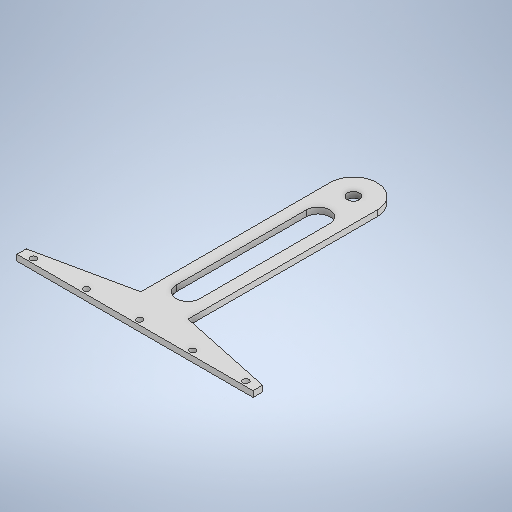
# Autodesk Inventor part: 03A
Saved by Autodesk Inventor 2025.1 (Build 291241000, 241)
## iProperties
Created: 2024-09-17
Part Number: 03A
Material: Generisch
Document SubType Name: Modeling
Designer: ffogue
Density: 1 g/cm^3
Appearance: Vorgabe
Author: ffogue
Autodesk Inventor part; units mm, degrees
ref_plane "YZ Plane" through (0, 0, 0) normal (1, 0, 0) x (0, 1, 0)
ref_plane "XZ Plane" through (0, 0, 0) normal (0, 1, 0) x (-1, 0, 0)
ref_plane "XY Plane" through (0, 0, 0) normal (0, 0, 1) x (1, 0, 0)
sketch "Sketch1" plane through (0, 0, 0) normal (0, 0, 1) x (1, 0, 0)
  line L0 (0, 0) -> (0, 91.5348) construction
  line L1 (-93.5855, 0) -> (93.5855, 0) construction
  arc A0 (20, 160) -> (-20, 160) centre (0, 160) ccw
  line L2 (-20, 160) -> (-20, 0)
  line L3 (-20, 0) -> (-100, -17)
  line L4 (-100, -17) -> (-100, -25)
  line L5 (-100, -25) -> (100, -25)
  line L6 (100, -25) -> (100, -17)
  line L7 (20, 160) -> (20, 0)
  line L8 (20, 0) -> (100, -17)
  dimension "d0" = 20
  dimension "d1" = 185
  dimension "d2" = 8
  dimension "d3" = 25
  dimension "d4" = 200
  constraints: 18 end point, 3 parallel, 3 perpendicular, 2 point on circle, 2 point on line, 2 tangent, 1 centre point, 1 horizontal, 1 midpoint, 1 vertical, 1 vertical alignment, 1 other
  measures "d0" radius of A0
  measures "d1" distance from line of L5 A0.centre
  measures "d2" distance of L3.end L4.end
  measures "d3" distance from line of L5 L2.end
  measures "d4" distance of L4.end L5.end
extrude "Extrusion1" add sketch "Sketch1" against normal blind 5
sketch "Sketch2" plane through (0, 0, 0) normal (0, 0, 1) x (1, 0, 0)
  line L0 (0, 20) -> (0, 130) construction
  line L1 (10, 20) -> (10, 130)
  line L2 (-10, 130) -> (-10, 20)
  arc A0 (-10, 20) -> (10, 20) centre (0, 20) ccw
  arc A1 (10, 130) -> (-10, 130) centre (0, 130) ccw
  arc A2 (20, 160) -> (-20, 160) centre (0, 160) ccw projected
  point P0 (0, 0)
  point P1 (0, 75)
  point P2 (0, 10)
  dimension "d7" = 30
  dimension "d8" = 10
  dimension "d9" = 110
  constraints: 8 end point, 5 point on circle, 4 tangent, 2 centre point, 1 midpoint, 1 parallel, 1 vertical, 1 vertical alignment
  measures "d7" distance of L0.end A2.centre
  measures "d8" radius of A0
  measures "d9" distance of L0.start L0.end
extrude "Extrusion2" cut sketch "Sketch2" against normal up to surface (5 mm away)
sketch "Sketch3" plane through (0, 0, 0) normal (0, 0, 1) x (1, 0, 0)
  line L0 (-100, -25) -> (100, -25) projected
  point P0 (0, 0)
  point P1 (-90, -21)
  point P2 (-45, -21)
  point P3 (0, -21)
  point P4 (45, -21)
  point P5 (90, -21)
  dimension "d12" = 45
  dimension "d13" = 45
  dimension "d14" = 45
  dimension "d15" = 45
  dimension "d16" = 4
  constraints: 4 horizontal alignment, 1 vertical alignment
  measures "d12" distance of point (-45, -21) point (-90, -21)
  measures "d13" distance of point (0, -21) point (-45, -21)
  measures "d14" distance of point (45, -21) point (0, -21)
  measures "d15" distance of point (90, -21) point (45, -21)
  measures "d16" distance from line of L0 point (-90, -21)
hole "Hole1" at (-90, -21, 0) at (-45, -21, 0) at (0, -21, 0) at (45, -21, 0) at (90, -21, 0) direction (0, 0, -1) diameter 5 depth 5
sketch "Sketch4" plane through (0, 0, 0) normal (0, 0, 1) x (1, 0, 0)
  arc A0 (20, 160) -> (-20, 160) centre (0, 160) ccw projected
  point P0 (0, 0)
  constraints: 1 coincident
hole "Hole2" at (0, 160, 0) direction (0, 0, -1) diameter 10 depth 5
equation "\"d13\" = d12"
equation "\"d14\" = d12"
equation "\"d15\" = d12"
body "Solid1"
